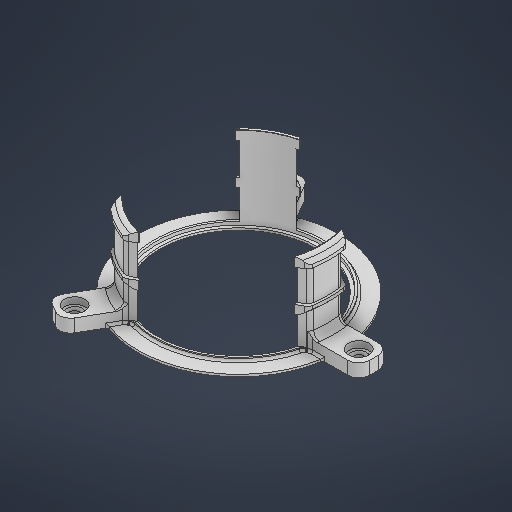
# Autodesk Inventor part: Adjustment_Base_Cap
Saved by Autodesk Inventor 2026.2 (Build 302298010, 298A)
## iProperties
Created: 2026-03-10
Part Number: Adjustment_Base_Cap
Material: Generic
Document SubType Name: Modeling
Designer: August
Density: 1 g/cm^3
Appearance: Default
Author: August
Autodesk Inventor part; units mm, degrees
ref_plane "YZ Plane" through (0, 0, 0) normal (1, 0, 0) x (0, 1, 0)
ref_plane "XZ Plane" through (0, 0, 0) normal (0, 1, 0) x (-1, 0, 0)
ref_plane "XY Plane" through (0, 0, 0) normal (0, 0, 1) x (1, 0, 0)
sketch "Sketch1" plane through (0, 0, 0) normal (0, 1, 0) x (-1, 0, 0)
  circle A0 centre (0, 0) radius 36.5
  circle A1 centre (0, 0) radius 38
  dimension "d0" = 73
  dimension "d1" = 76
  constraints: 2 centre point, 2 coincident
  measures "d0" diameter of A0
  measures "d1" diameter of A1
extrude "Extrusion1" add sketch "Sketch1" along normal blind 1
sketch "Sketch2" plane through (0, 0, 0) normal (0, 1, 0) x (-1, 0, 0)
  circle A0 centre (0, 0) radius 38
  circle A1 centre (0, 0) radius 39
  dimension "d4" = 76
  dimension "d5" = 78
  constraints: 2 centre point, 2 coincident
  measures "d4" diameter of A0
  measures "d5" diameter of A1
extrude "Extrusion2" add sketch "Sketch2" along normal blind 2.5
sketch "Sketch4" plane through (0, 0, 0) normal (0, 1, 0) x (-1, 0, 0)
  line L0 (0, 0) -> (-60.4929, 0)
  line L1 (0, 0) -> (-59.5739, 10.5045)
  line L2 (0, 0) -> (-59.5739, -10.5045)
  circle A0 centre (0, 0) radius 38
  circle A1 centre (0, 0) radius 40.9
  line L3 (-40.2786, 7.1022) -> (-36.7799, 9.5521)
  line L4 (-40.2786, -7.1022) -> (-36.7799, -9.5521)
  dimension "d10" = 20
  dimension "d12" = 76
  dimension "d13" = 81.8
  dimension "d14" = 45
  dimension "d15" = 45
  constraints: 10 end point, 4 point on circle, 3 coincident, 2 centre point, 2 point on line, 1 horizontal, 6 other
  measures "d12" diameter of A0
  measures "d13" diameter of A1
  measures "d14" angle of L1 L3
  measures "d15" angle of L2 L4
extrude "Extrusion3" add sketch "Sketch4" along normal blind 35.75 contours A0 L2 A1 L0 | L0 A1 L1 A0 | L1 L3 A0 | A0 L4 L2
sketch "Sketch5" plane through (0, 0, 0) normal (0, 0, 1) x (1, 0, 0)
  line L0 (0, 0) -> (38, 0)
  line L1 (38, 0) -> (38, 20)
  line L2 (38, 20) -> (42, 20)
  line L3 (42, 20) -> (42, 18.5)
  line L4 (42, 18.5) -> (49.0711, 18.5) construction
  line L5 (38, 20) -> (38, 35)
  line L6 (38, 35) -> (42, 35)
  line L7 (42, 35) -> (42, 36.5)
  line L8 (38, 35) -> (38, 39)
  line L9 (38, 39) -> (39.5, 39)
  line L10 (42, 36.5) -> (39.5, 39)
  line L11 (0, -7.8) -> (0, 46.8) projected
  line L12 (38, 20) -> (38, 16)
  line L13 (38, 16) -> (39.5, 16)
  line L14 (39.5, 16) -> (42, 18.5)
  point P0 (38, 13)
  point P1 (42.5, 18.5)
  dimension "d18" = 38
  dimension "d19" = 20
  dimension "d20" = 4
  dimension "d23" = 15
  dimension "d24" = 1.5
  dimension "d26" = 4
  dimension "d27" = 4
  dimension "d28" = 135
  dimension "d40" = 4
  dimension "d41" = 1.5
  dimension "d42" = 135
  constraints: 28 end point, 7 perpendicular, 3 horizontal, 2 point on line, 1 vertical
  measures "d18" distance of L0.start L0.end
  measures "d19" distance of L0.end L1.end
  measures "d20" distance of L1.end L2.end
  measures "d23" distance of L1.end L5.end
  measures "d24" distance of L6.end L7.end
  measures "d26" distance of L5.end L6.end
  measures "d27" distance of L5.end L8.end
  measures "d28" angle of L10 L7
  measures "d40" distance of L1.end L12.end
  measures "d41" distance of L12.end L13.end
  measures "d42" angle of L3 L14
revolve "Revolution1" add sketch "Sketch5" angle 33 mid plane about axis through (0, -10, 0) along (0, 1, 0)
sketch "Sketch6" plane through (0, 39, 0) normal (0, 1, 0) x (1, 0, 0)
  circle A0 centre (0, 0) radius 43.5
  circle A1 centre (0, 0) radius 38.5
  line L0 (0, 0) -> (62.3795, 0)
  line L1 (0, 0) -> (59.8107, 17.7167)
  line L2 (0, 0) -> (59.8107, -17.7167)
  line L3 (36.9146, -10.9346) -> (42.8067, -7.7354)
  line L4 (36.9146, 10.9346) -> (42.8067, 7.7354)
  point P0 (0, 0)
  point P1 (41.7087, 12.3547)
  point P2 (41.7087, -12.3547)
  dimension "d30" = 77
  dimension "d33" = 33
  dimension "d35" = 87
  dimension "d36" = 45
  dimension "d37" = 45
  constraints: 10 end point, 4 point on circle, 2 centre point, 2 coincident, 2 point on line, 1 horizontal, 7 other
  measures "d30" diameter of A1
  measures "d35" diameter of A0
  measures "d36" angle of L2 L3
  measures "d37" angle of L1 L4
extrude "Extrusion4" cut sketch "Sketch6" against normal blind 28 contours L4 L1 A0 | A0 L2 L3
fillet "Fillet1" radius 3 10 edges at (41.0967, 35.75, 8.6639) (40.2786, 27.5, 7.1022) (41.0967, 19.25, 8.6639) (41.0967, 19.25, -8.6639) (41.0967, 35.75, -8.6639) (40.2786, 27.5, -7.1022) (40.2786, 8.7, -7.1022) (40.2786, 8.7, 7.1022) (38.0211, 1.25, 8.6829) (38.0211, 1.25, -8.6829)
fillet "Fillet2" radius 3 3 edges at (38.3977, 16, 9.2666) (38.3977, 16, -9.2666) (39.5, 39, 0)
sketch "Sketch7" plane through (0, 0, 0) normal (0, -1, 0) x (1, 0, 0)
  circle A0 centre (0, 0) radius 46.5
  line L0 (46.5, 0) -> (48.5, 0)
  line L1 (48.5, 0) -> (55.5, 0)
  circle A1 centre (55.5, 0) radius 2.5
  line L2 (55.5, 7) -> (62.5, 7)
  line L3 (62.5, 7) -> (62.5, 0)
  line L4 (55.5, -7) -> (62.5, -7)
  line L5 (62.5, -7) -> (62.5, 0)
  line L6 (55.5, -7) -> (45.9701, -7)
  line L7 (55.5, 7) -> (45.9701, 7)
  circle A2 centre (0, 0) radius 44.5
  circle A3 centre (0, 0) radius 39.5
  line L8 (45.9701, 7) -> (38.8748, 7)
  line L9 (45.9701, -7) -> (38.8748, -7)
  dimension "d46" = 2
  dimension "d47" = 7
  dimension "d48" = 7
  dimension "d49" = 5
  dimension "d50" = 7
  dimension "d51" = 7
  dimension "d52" = 89
  dimension "d54" = 2
  dimension "d55" = 7
  dimension "d56" = 7
  dimension "d59" = 79
  constraints: 20 end point, 5 point on circle, 5 point on line, 4 centre point, 4 coincident, 2 horizontal, 2 parallel, 2 perpendicular, 1 line through centre
  measures "d46" distance of L0.start L0.end
  measures "d47" distance of L0.end L1.end
  measures "d48" distance of L1.end L3.end
  measures "d49" diameter of A1
  measures "d50" distance of A1.centre L2.start
  measures "d51" distance of A1.centre L4.start
  measures "d52" diameter of A2
  measures "d54" radial gap between concentric circles of A0 A2
  measures "d55" distance of L2.end L3.end
  measures "d56" distance of L4.end L3.end
  measures "d59" diameter of A3
extrude "Extrusion5" add sketch "Sketch7" against normal blind 6 contours A0 L9 A2 L8 | A0 L7 L2 L3 L5 L4 L6 | A2 L9 A3 L8 picked at (44.7232, 6.2258) picked at (40.6808, 6.2268)
sketch "Sketch8" plane through (0, 6, 0) normal (0, 1, 0) x (1, 0, 0)
  line L0 (0, 0) -> (55.5, 0)
  circle A0 centre (55.5, 0) radius 4.75
  dimension "d60" = 55.5
  dimension "d61" = 9.5
  constraints: 2 end point, 1 centre point, 1 coincident, 1 horizontal
  measures "d60" distance of L0.start L0.end
  measures "d61" diameter of A0
extrude "Extrusion6" cut sketch "Sketch8" against normal blind 3
sketch "Sketch9" plane through (0, 0, 0) normal (0, 1, 0) x (-1, 0, 0)
  circle A0 centre (0, 0) radius 39
  circle A1 centre (0, 0) radius 44.5
  circle A2 centre (0, 0) radius 46.5
  dimension "d64" = 78
  dimension "d65" = 89
  dimension "d66" = 2
  constraints: 3 centre point, 3 coincident
  measures "d64" diameter of A0
  measures "d65" diameter of A1
  measures "d66" radial gap between concentric circles of A2 A1
extrude "Extrusion7" add sketch "Sketch9" along normal blind 1 contours A1 | A2
fillet "Fillet3" radius 3 5 edges at (40.038, 3.5, 7) (40.3273, 6, -6.4237) (40.3273, 6, 6.4237) (40.9, 6, 0) (40.038, 3.5, -7)
fillet "Fillet4" radius 5 2 edges at (62.5, 3, 7) (62.5, 3, -7)
fillet "Fillet5" radius 1 1 edges at (53, 3, 0)
pattern_circular "Circular Pattern1" count 3 over 360 about axis through (0, -10, 0) along (0, 1, 0) of "Fillet5", "Fillet4", "Fillet3", "Extrusion6", "Extrusion5", "Fillet2", "Fillet1", "Extrusion3", "Extrusion4", "Revolution1"
fillet "Fillet6" radius 1 39 edges at (38.2031, 1, 8.7823) (39.0928, 1, 7.9325) (39.334, 1, 7.7607) (40.3226, 1, 7.1769) (43.6538, 1, 7) (-11.4958, 1, 37.476) (-12.6766, 1, 37.8216) (-12.946, 1, 37.9446) (-13.9459, 1, 38.5088) (-15.7647, 1, 41.3053) (19.5, 1, 33.775) (-11.4958, 1, -37.476) (-12.6766, 1, -37.8216) (-12.946, 1, -37.9446) (-13.9459, 1, -38.5088) (-15.7647, 1, -41.3053) (38.2031, 1, -8.7823) (39.0928, 1, -7.9325) (39.334, 1, -7.7607) (40.3226, 1, -7.1769) (43.6538, 1, -7) (19.5, 1, -33.775) (45.9701, 0.5, 7) (45.9701, 0.5, -7) (-16.9229, 0.5, -43.3113) (-26.3767, 1, -31.3319) (-26.388, 1, -30.1839) (-26.4162, 1, -29.8891) (-26.7072, 1, -28.6937) (-39, 1, 0) (-26.7072, 1, 28.6937) (-26.4162, 1, 29.8891) (-26.388, 1, 30.1839) (-26.3767, 1, 31.3319) (-27.8891, 1, 34.3053) (-27.8891, 1, -34.3053) (-29.0472, 0.5, -36.3113) (-29.0472, 0.5, 36.3113) (-16.9229, 0.5, 43.3113)
body "Solid1"
